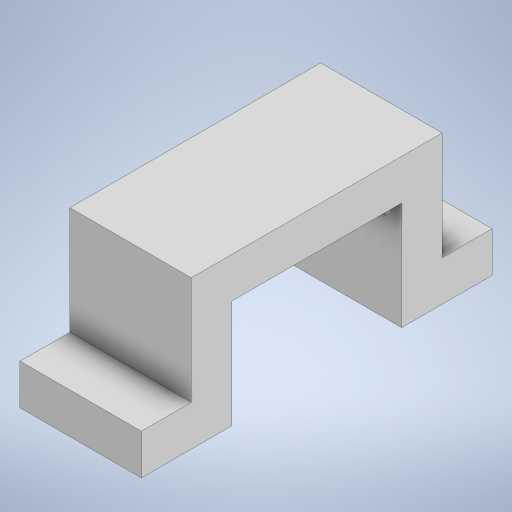
# Autodesk Inventor part: motor_bracket
Saved by Autodesk Inventor 2023 (Build 270158000, 158)
## iProperties
Created: 2024-04-04
Part Number: motor_bracket
Material: Ogólny
Document SubType Name: Modeling
Designer: Kamil
Density: 1 g/cm^3
Appearance: Domyślna
Author: Kamil
Autodesk Inventor part; units mm, degrees
ref_plane "YZ Plane" through (0, 0, 0) normal (1, 0, 0) x (0, 1, 0)
ref_plane "XZ Plane" through (0, 0, 0) normal (0, 1, 0) x (-1, 0, 0)
ref_plane "XY Plane" through (0, 0, 0) normal (0, 0, 1) x (1, 0, 0)
sketch "Szkic1" plane through (0, 0, 0) normal (1, 0, 0) x (0, 1, 0)
  line L0 (-4, 6.3) -> (4, 6.3)
  line L1 (4, 6.3) -> (4, -6.3)
  line L2 (4, -6.3) -> (-4, -6.3)
  line L3 (-4, 6.3) -> (-4, 13)
  line L4 (-4, -6.3) -> (-4, -13)
  line L5 (-1, -13) -> (-1, -9.3)
  line L6 (-1, -9.3) -> (7, -9.3)
  line L7 (7, -9.3) -> (7, 9.3)
  line L8 (7, 9.3) -> (-1, 9.3)
  line L9 (-1, 9.3) -> (-1, 13)
  line L10 (-4, 13) -> (-1, 13)
  line L11 (-4, -13) -> (-1, -13)
  point P0 (0, 0)
  point P1 (0, 6.3)
  point P2 (4, 0)
  dimension "d0" = 8
  dimension "d1" = 12.6
  dimension "d2" = 6.7
  dimension "d3" = 6.7
  dimension "d4" = 3
  constraints: 24 end point, 3 parallel, 2 collinear, 2 horizontal, 2 midpoint, 2 perpendicular, 2 vertical, 1 horizontal alignment, 1 vertical alignment, 4 other
  measures "d0" distance of L1.end L2.end
  measures "d1" distance of L0.end L1.end
  measures "d2" distance of L0.start L3.end
  measures "d3" distance of L2.end L4.end
  measures "d4" distance between parallel lines of L0 L8
extrude "Wyciągnięcie proste1" add sketch "Szkic1" along normal blind 9
sketch "Szkic2" plane through (0, 4, -6.3) normal (0, -1, 0) x (1, 0, 0)
  line L0 (0, 12.6) -> (0, 0) projected
  line L1 (0, 0) -> (9, 0) projected
  line L2 (9, 12.6) -> (9, 0) projected
  line L3 (0, 12.6) -> (9, 12.6) projected
  line L4 (8.2, 12.6) -> (8.2, 0)
  line L5 (4, 12.6) -> (4, 0)
  line L6 (3.2, 12.6) -> (3.2, 0)
  line L7 (0.8, 0) -> (0.8, 12.6)
  line L8 (0.8, 12.6) -> (3.2, 12.6)
  line L9 (3.2, 12.6) -> (3.2, 11.8)
  line L10 (3.2, 11.8) -> (0.8, 11.8)
  line L11 (0.8, 11.8) -> (0.8, 12.6)
  line L12 (0.8, 0) -> (3.2, 0)
  line L13 (3.2, 0) -> (3.2, 0.8)
  line L14 (3.2, 0.8) -> (0.8, 0.8)
  line L15 (0.8, 0.8) -> (0.8, 0)
  line L16 (4, 12.6) -> (8.2, 12.6)
  line L17 (8.2, 12.6) -> (8.2, 11.8)
  line L18 (8.2, 11.8) -> (4, 11.8)
  line L19 (4, 11.8) -> (4, 12.6)
  line L20 (4, 0) -> (8.2, 0)
  line L21 (8.2, 0) -> (8.2, 0.8)
  line L22 (8.2, 0.8) -> (4, 0.8)
  line L23 (4, 0.8) -> (4, 0)
  point P0 (0, 6.3)
  point P1 (4, 0.8)
  point P2 (0.8, 0.8)
  point P3 (0.8, 11.8)
  dimension "d7" = 0.8
  dimension "d8" = 4.2
  dimension "d9" = 0.8
  dimension "d10" = 2.4
  dimension "d11" = 0.8
  dimension "d12" = 0.8
  dimension "d13" = 0.8
  dimension "d14" = 0.8
  constraints: 40 end point, 12 point on line, 8 parallel, 8 perpendicular, 4 horizontal
  measures "d7" distance between parallel lines of L2 L4
  measures "d8" distance between parallel lines of L4 L5
  measures "d9" distance between parallel lines of L5 L6
  measures "d10" distance between parallel lines of L6 L7
  measures "d11" distance between parallel lines of L3 L10
  measures "d12" distance between parallel lines of L1 L14
  measures "d13" distance between parallel lines of L16 L18
  measures "d14" distance between parallel lines of L1 L22
extrude "Wyciągnięcie proste2" add sketch "Szkic2" along normal blind 0.5 contours L3 L6 L10 L7 | L7 L14 L6 L1 | L3 L4 L18 L5 | L5 L22 L4 L1
sketch "Szkic3" plane through (0, 3.5, -6.3) normal (0, -1, 0) x (1, 0, 0)
  line L0 (8.2, 11.8) -> (8.2, 12.6) projected
  line L1 (4, 12.6) -> (8.2, 12.6) projected
  line L2 (4, 12.6) -> (4, 11.8) projected
  line L3 (4, 11.8) -> (8.2, 11.8) projected
  line L4 (3.2, 11.8) -> (3.2, 12.6) projected
  line L5 (0.8, 12.6) -> (3.2, 12.6) projected
  line L6 (0.8, 12.6) -> (0.8, 11.8) projected
  line L7 (0.8, 11.8) -> (3.2, 11.8) projected
  line L8 (0.8, 0.8) -> (0.8, 0) projected
  line L9 (3.2, 0) -> (0.8, 0) projected
  line L10 (3.2, 0) -> (3.2, 0.8) projected
  line L11 (3.2, 0.8) -> (0.8, 0.8) projected
  line L12 (4, 0.8) -> (4, 0) projected
  line L13 (8.2, 0) -> (4, 0) projected
  line L14 (8.2, 0) -> (8.2, 0.8) projected
  line L15 (8.2, 0.8) -> (4, 0.8) projected
  line L16 (8.2, 12.6) -> (8.2, 11.8) projected
  line L17 (8.2, 12.2) -> (0.8, 12.2)
  line L18 (8.2, 0.4) -> (0.8, 0.4)
  point P0 (0, 6.3)
  point P1 (4, 0.4)
  point P2 (3.2, 0.4)
  point P3 (4, 12.2)
  point P4 (3.2, 12.2)
  constraints: 4 end point, 4 midpoint
extrude "Wyciągnięcie proste3" add sketch "Szkic3" along normal blind 0.5 contours L17 L2 L1 L0 | L17 L6 L5 L4 | L18 L10 L9 L8 | L18 L14 L13 L12
